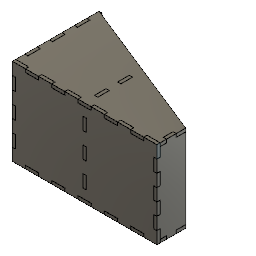
verkefni2_box (Autodesk Fusion 360 design; units mm, degrees)
Autodesk Fusion 360 part; units mm, degrees
sketch "Sketch1" plane through (0, 0, 0) normal (0, 0, 1) x (1, 0, 0)
  line L0 (0, 0) -> (125, 0)
  line L1 (125, 0) -> (125, 75)
  line L2 (125, 75) -> (0, 75)
  line L3 (0, 75) -> (0, 0)
  dimension "d18" = 125
  dimension "d19" = 75
  constraint horizontal L0
  constraint vertical L1
  constraint horizontal L2
  constraint vertical L3
  constraint coincident L0.start L3.end
  measures "d18" distance of L0.start L0.end
  measures "d19" distance of L0.start L2.end
extrude "Extrude1" add sketch "Sketch1" against normal blind 2.8 makes body 1
sketch "Sketch3" plane through (0, 0, 0) normal (-1, 0, 0) x (0, 0, 1)
  line L0 (0, 0) -> (0, 75)
  line L1 (0, 75) -> (-2.8, 75)
  line L2 (-2.8, 75) -> (-2.8, 0)
  line L3 (-2.8, 0) -> (0, 0)
  line L4 (0, 10.7143) -> (-2.8, 10.7143)
  line L5 (-2.8, 10.7143) -> (-2.8, 21.4286)
  line L6 (-2.8, 21.4286) -> (0, 21.4286)
  line L7 (0, 21.4286) -> (0, 10.7143)
  dimension "d24" = 10.7143
  dimension "d25" = 10.7143
  constraint horizontal L4
  constraint vertical L5
  constraint horizontal L6
  constraint vertical L7
  constraint coincident L2 L5.end
  constraint coincident L0 L4.start
  measures "d24" distance of L4.start L6.end
  measures "d25" distance of L0.start L4
extrude "Extrude2" cut sketch "Sketch3" against normal blind 2.8 contours L0 L2 L4 L5 L6 L7 bodies 1
pattern_linear "R-Pattern1" count 3 spacing 21.4286 along (0, 1, 0) of "Extrude2"
sketch "Sketch4" plane through (125, 0, 0) normal (1, 0, 0) x (0, 0, -1)
  line L0 (0, 75) -> (0, 0)
  line L1 (0, 0) -> (2.8, 0)
  line L2 (2.8, 0) -> (2.8, 75)
  line L3 (2.8, 75) -> (0, 75)
  line L4 (2.8, 10.7143) -> (0, 10.7143)
  line L5 (0, 10.7143) -> (0, 21.4286)
  line L6 (0, 21.4286) -> (2.8, 21.4286)
  line L7 (2.8, 21.4286) -> (2.8, 10.7143)
  dimension "d32" = 10.7143
  dimension "d33" = 10.7143
  constraint horizontal L4
  constraint vertical L5
  constraint horizontal L6
  constraint vertical L7
  constraint coincident L0 L5.end
  constraint coincident L2 L4.start
  measures "d32" distance of L4.end L5.end
  measures "d33" distance of L0.end L4
extrude "Extrude3" cut sketch "Sketch4" against normal blind 2.8 contours L0 L2 L4 L5 L6 L7 bodies 1
pattern_linear "R-Pattern2" count 3 spacing 21.4286 along (0, 1, 0) of "Extrude3"
sketch "Sketch5" plane through (0, 0, 0) normal (0, -1, 0) x (1, 0, 0)
  line L0 (125, 0) -> (0, 0)
  line L1 (0, 0) -> (0, -2.8)
  line L2 (0, -2.8) -> (125, -2.8)
  line L3 (125, -2.8) -> (125, 0)
  line L4 (11.3636, 0) -> (22.7273, 0)
  line L5 (22.7273, 0) -> (22.7273, -2.8)
  line L6 (22.7273, -2.8) -> (11.3636, -2.8)
  line L7 (11.3636, -2.8) -> (11.3636, 0)
  dimension "d40" = 11.3636
  dimension "d41" = 11.3636
  constraint horizontal L4
  constraint vertical L5
  constraint horizontal L6
  constraint vertical L7
  constraint coincident L2 L5.end
  constraint coincident L0 L4.start
  measures "d40" distance of L5.end L6.end
  measures "d41" horizontal distance of L0.end L6.end
extrude "Extrude4" cut sketch "Sketch5" against normal blind 2.8 contours L0 L2 L4 L5 L6 L7 bodies 1
pattern_linear "R-Pattern3" count 5 spacing 22.7273 along (1, 0, 0) of "Extrude4"
sketch "Sketch6" plane through (0, 75, 0) normal (0, 1, 0) x (-1, 0, 0)
  line L0 (0, 0) -> (-125, 0)
  line L1 (-125, 0) -> (-125, -2.8)
  line L2 (-125, -2.8) -> (0, -2.8)
  line L3 (0, -2.8) -> (0, 0)
  line L4 (-11.3636, -2.8) -> (-22.7273, -2.8)
  line L5 (-22.7273, -2.8) -> (-22.7273, 0)
  line L6 (-22.7273, 0) -> (-11.3636, 0)
  line L7 (-11.3636, 0) -> (-11.3636, -2.8)
  dimension "d48" = 11.3636
  dimension "d49" = 11.3636
  constraint horizontal L4
  constraint vertical L5
  constraint horizontal L6
  constraint vertical L7
  constraint coincident L0 L5.end
  constraint coincident L2 L4.start
  measures "d48" distance of L4.start L4.end
  measures "d49" distance of L0.start L6.end
extrude "Extrude5" cut sketch "Sketch6" against normal blind 2.8 contours L0 L2 L4 L5 L6 L7 bodies 1
pattern_linear "R-Pattern4" count 5 spacing 22.7273 along (1, 0, 0) of "Extrude5"
sketch "Sketch7" plane through (0, 0, -2.8) normal (0, 0, -1) x (-1, 0, 0)
  line L0 (-102.2727, 75) -> (-102.2727, 72.2)
  line L1 (-102.2727, 72.2) -> (-113.6364, 72.2)
  line L2 (-113.6364, 72.2) -> (-113.6364, 75)
  line L3 (-113.6364, 75) -> (-125, 75)
  line L4 (-125, 75) -> (-125, 64.2857)
  line L5 (-125, 64.2857) -> (-122.2, 64.2857)
  line L6 (-122.2, 64.2857) -> (-122.2, 53.5714)
  line L7 (-122.2, 53.5714) -> (-125, 53.5714)
  line L8 (-125, 53.5714) -> (-125, 42.8571)
  line L9 (-125, 42.8571) -> (-122.2, 42.8571)
  line L10 (-122.2, 42.8571) -> (-122.2, 32.1429)
  line L11 (-122.2, 32.1429) -> (-125, 32.1429)
  line L12 (-125, 32.1429) -> (-125, 21.4286)
  line L13 (-125, 21.4286) -> (-122.2, 21.4286)
  line L14 (-122.2, 21.4286) -> (-122.2, 10.7143)
  line L15 (-122.2, 10.7143) -> (-125, 10.7143)
  line L16 (-125, 10.7143) -> (-125, 0)
  line L17 (-125, 0) -> (-113.6364, 0)
  line L18 (-113.6364, 0) -> (-113.6364, 2.8)
  line L19 (-113.6364, 2.8) -> (-102.2727, 2.8)
  line L20 (-102.2727, 2.8) -> (-102.2727, 0)
  line L21 (-102.2727, 0) -> (-90.9091, 0)
  line L22 (-90.9091, 0) -> (-90.9091, 2.8)
  line L23 (-90.9091, 2.8) -> (-79.5455, 2.8)
  line L24 (-79.5455, 2.8) -> (-79.5455, 0)
  line L25 (-79.5455, 0) -> (-68.1818, 0)
  line L26 (-68.1818, 0) -> (-68.1818, 2.8)
  line L27 (-68.1818, 2.8) -> (-56.8182, 2.8)
  line L28 (-56.8182, 2.8) -> (-56.8182, 0)
  line L29 (-56.8182, 0) -> (-45.4545, 0)
  line L30 (-45.4545, 0) -> (-45.4545, 2.8)
  line L31 (-45.4545, 2.8) -> (-34.0909, 2.8)
  line L32 (-34.0909, 2.8) -> (-34.0909, 0)
  line L33 (-34.0909, 0) -> (-22.7273, 0)
  line L34 (-22.7273, 0) -> (-22.7273, 2.8)
  line L35 (-22.7273, 2.8) -> (-11.3636, 2.8)
  line L36 (-11.3636, 2.8) -> (-11.3636, 0)
  line L37 (-11.3636, 0) -> (0, 0)
  line L38 (0, 0) -> (0, 10.7143)
  line L39 (0, 10.7143) -> (-2.8, 10.7143)
  line L40 (-2.8, 10.7143) -> (-2.8, 21.4286)
  line L41 (-2.8, 21.4286) -> (0, 21.4286)
  line L42 (0, 21.4286) -> (0, 32.1429)
  line L43 (0, 32.1429) -> (-2.8, 32.1429)
  line L44 (-2.8, 32.1429) -> (-2.8, 42.8571)
  line L45 (-2.8, 42.8571) -> (0, 42.8571)
  line L46 (0, 42.8571) -> (0, 53.5714)
  line L47 (0, 53.5714) -> (-2.8, 53.5714)
  line L48 (-2.8, 53.5714) -> (-2.8, 64.2857)
  line L49 (-2.8, 64.2857) -> (0, 64.2857)
  line L50 (0, 64.2857) -> (0, 75)
  line L51 (0, 75) -> (-11.3636, 75)
  line L52 (-11.3636, 75) -> (-11.3636, 72.2)
  line L53 (-11.3636, 72.2) -> (-22.7273, 72.2)
  line L54 (-22.7273, 72.2) -> (-22.7273, 75)
  line L55 (-22.7273, 75) -> (-34.0909, 75)
  line L56 (-34.0909, 75) -> (-34.0909, 72.2)
  line L57 (-34.0909, 72.2) -> (-45.4545, 72.2)
  line L58 (-45.4545, 72.2) -> (-45.4545, 75)
  line L59 (-45.4545, 75) -> (-56.8182, 75)
  line L60 (-56.8182, 75) -> (-56.8182, 72.2)
  line L61 (-56.8182, 72.2) -> (-68.1818, 72.2)
  line L62 (-68.1818, 72.2) -> (-68.1818, 75)
  line L63 (-68.1818, 75) -> (-79.5455, 75)
  line L64 (-79.5455, 75) -> (-79.5455, 72.2)
  line L65 (-79.5455, 72.2) -> (-90.9091, 72.2)
  line L66 (-90.9091, 72.2) -> (-90.9091, 75)
  line L67 (-90.9091, 75) -> (-102.2727, 75)
  line L68 (0, 0) -> (-61.1, 0)
  line L69 (-61.1, 0) -> (-61.1, 75)
  line L70 (-61.1, 0) -> (-63.9, 0)
  line L71 (-63.9, 0) -> (-63.9, 75)
  line L72 (-63.9, 75) -> (-61.1, 75)
  line L73 (-61.1, 75) -> (-61.1, 0)
  line L74 (-61.1, 10.7143) -> (-63.9, 10.7143)
  line L75 (-63.9, 10.7143) -> (-63.9, 21.4286)
  line L76 (-63.9, 21.4286) -> (-61.1, 21.4286)
  line L77 (-61.1, 21.4286) -> (-61.1, 10.7143)
  dimension "d56" = 61.1
  dimension "d57" = 75
  dimension "d58" = 2.8
  dimension "d59" = 75
  dimension "d60" = 10.7143
  dimension "d61" = 10.7143
  constraint coincident L37.end L38.start
  constraint perpendicular L28 L68
  constraint perpendicular L61 L69
  constraint horizontal L70
  constraint vertical L71
  constraint horizontal L72
  constraint vertical L73
  constraint horizontal L74
  constraint vertical L75
  constraint horizontal L76
  constraint vertical L77
  constraint coincident L71 L75.end
  constraint coincident L69 L74.start
  measures "d56" distance of L37.end L68.end
  measures "d57" distance of L68.end L69.end
  measures "d58" distance of L68.end L70.end
  measures "d59" distance of L68.end L69.end
  measures "d60" distance of L70 L74
  measures "d61" distance of L74.end L75.end
extrude "Extrude6" cut sketch "Sketch7" against normal blind 2.8 contours L69 L71 L73 L74 L75 L76 L77 bodies 1
pattern_linear "R-Pattern5" count 3 spacing 21.4286 along (0, 1, 0) of "Extrude6"
sketch "Sketch10" plane through (0, 0, -2.8) normal (0, 0, -1) x (-1, 0, 0)
  line L0 (-63.9, 53.5714) -> (-63.9, 64.2857)
  line L1 (-63.9, 64.2857) -> (-61.1, 64.2857)
  line L2 (-61.1, 64.2857) -> (-61.1, 53.5714)
  line L3 (-61.1, 53.5714) -> (-63.9, 53.5714)
  line L4 (-63.9, 32.1429) -> (-63.9, 42.8571)
  line L5 (-63.9, 42.8571) -> (-61.1, 42.8571)
  line L6 (-61.1, 42.8571) -> (-61.1, 32.1429)
  line L7 (-61.1, 32.1429) -> (-63.9, 32.1429)
  line L8 (-63.9, 10.7143) -> (-63.9, 21.4286)
  line L9 (-63.9, 21.4286) -> (-61.1, 21.4286)
  line L10 (-61.1, 21.4286) -> (-61.1, 10.7143)
  line L11 (-61.1, 10.7143) -> (-63.9, 10.7143)
  line L12 (-102.2727, 75) -> (-102.2727, 72.2)
  line L13 (-102.2727, 72.2) -> (-113.6364, 72.2)
  line L14 (-113.6364, 72.2) -> (-113.6364, 75)
  line L15 (-113.6364, 75) -> (-125, 75)
  line L16 (-125, 75) -> (-125, 64.2857)
  line L17 (-125, 64.2857) -> (-122.2, 64.2857)
  line L18 (-122.2, 64.2857) -> (-122.2, 53.5714)
  line L19 (-122.2, 53.5714) -> (-125, 53.5714)
  line L20 (-125, 53.5714) -> (-125, 42.8571)
  line L21 (-125, 42.8571) -> (-122.2, 42.8571)
  line L22 (-122.2, 42.8571) -> (-122.2, 32.1429)
  line L23 (-122.2, 32.1429) -> (-125, 32.1429)
  line L24 (-125, 32.1429) -> (-125, 21.4286)
  line L25 (-125, 21.4286) -> (-122.2, 21.4286)
  line L26 (-122.2, 21.4286) -> (-122.2, 10.7143)
  line L27 (-122.2, 10.7143) -> (-125, 10.7143)
  line L28 (-125, 10.7143) -> (-125, 0)
  line L29 (-125, 0) -> (-113.6364, 0)
  line L30 (-113.6364, 0) -> (-113.6364, 2.8)
  line L31 (-113.6364, 2.8) -> (-102.2727, 2.8)
  line L32 (-102.2727, 2.8) -> (-102.2727, 0)
  line L33 (-102.2727, 0) -> (-90.9091, 0)
  line L34 (-90.9091, 0) -> (-90.9091, 2.8)
  line L35 (-90.9091, 2.8) -> (-79.5455, 2.8)
  line L36 (-79.5455, 2.8) -> (-79.5455, 0)
  line L37 (-79.5455, 0) -> (-68.1818, 0)
  line L38 (-68.1818, 0) -> (-68.1818, 2.8)
  line L39 (-68.1818, 2.8) -> (-56.8182, 2.8)
  line L40 (-56.8182, 2.8) -> (-56.8182, 0)
  line L41 (-56.8182, 0) -> (-45.4545, 0)
  line L42 (-45.4545, 0) -> (-45.4545, 2.8)
  line L43 (-45.4545, 2.8) -> (-34.0909, 2.8)
  line L44 (-34.0909, 2.8) -> (-34.0909, 0)
  line L45 (-34.0909, 0) -> (-22.7273, 0)
  line L46 (-22.7273, 0) -> (-22.7273, 2.8)
  line L47 (-22.7273, 2.8) -> (-11.3636, 2.8)
  line L48 (-11.3636, 2.8) -> (-11.3636, 0)
  line L49 (-11.3636, 0) -> (0, 0)
  line L50 (0, 0) -> (0, 10.7143)
  line L51 (0, 10.7143) -> (-2.8, 10.7143)
  line L52 (-2.8, 10.7143) -> (-2.8, 21.4286)
  line L53 (-2.8, 21.4286) -> (0, 21.4286)
  line L54 (0, 21.4286) -> (0, 32.1429)
  line L55 (0, 32.1429) -> (-2.8, 32.1429)
  line L56 (-2.8, 32.1429) -> (-2.8, 42.8571)
  line L57 (-2.8, 42.8571) -> (0, 42.8571)
  line L58 (0, 42.8571) -> (0, 53.5714)
  line L59 (0, 53.5714) -> (-2.8, 53.5714)
  line L60 (-2.8, 53.5714) -> (-2.8, 64.2857)
  line L61 (-2.8, 64.2857) -> (0, 64.2857)
  line L62 (0, 64.2857) -> (0, 75)
  line L63 (0, 75) -> (-11.3636, 75)
  line L64 (-11.3636, 75) -> (-11.3636, 72.2)
  line L65 (-11.3636, 72.2) -> (-22.7273, 72.2)
  line L66 (-22.7273, 72.2) -> (-22.7273, 75)
  line L67 (-22.7273, 75) -> (-34.0909, 75)
  line L68 (-34.0909, 75) -> (-34.0909, 72.2)
  line L69 (-34.0909, 72.2) -> (-45.4545, 72.2)
  line L70 (-45.4545, 72.2) -> (-45.4545, 75)
  line L71 (-45.4545, 75) -> (-56.8182, 75)
  line L72 (-56.8182, 75) -> (-56.8182, 72.2)
  line L73 (-56.8182, 72.2) -> (-68.1818, 72.2)
  line L74 (-68.1818, 72.2) -> (-68.1818, 75)
  line L75 (-68.1818, 75) -> (-79.5455, 75)
  line L76 (-79.5455, 75) -> (-79.5455, 72.2)
  line L77 (-79.5455, 72.2) -> (-90.9091, 72.2)
  line L78 (-90.9091, 72.2) -> (-90.9091, 75)
  line L79 (-90.9091, 75) -> (-102.2727, 75)
  line L80 (0, 0) -> (-61.1, 0)
  line L81 (-61.1, 0) -> (-63.9, 0)
  line L82 (-63.9, 0) -> (-63.9, 75)
  line L83 (-63.9, 75) -> (-61.1, 75)
  line L84 (-61.1, 75) -> (-61.1, 0)
  dimension "d72" = 61.1
  dimension "d73" = 2.8
  dimension "d74" = 75
  constraint coincident L49.end L50.start
  constraint perpendicular L50 L80
  constraint horizontal L81
  constraint vertical L82
  constraint horizontal L83
  constraint vertical L84
  measures "d72" distance of L49.end L80.end
  measures "d73" distance of L80.end L81.end
  measures "d74" distance of L80.end L83.end
extrude "Extrude7" add sketch "Sketch10" along normal blind 47.2 separate body contours L0 L1 L2 L3 L82 L84 | L3 L5 L82 L84 | L1 L73 L82 L84 | L4 L5 L6 L7 L82 L84 | L73 L82 L83 L84 | L7 L9 L82 L84 | L8 L9 L10 L11 L82 L84 | L11 L39 L82 L84 | L39 L81 L82 L84 makes body 2
sketch "Sketch12" plane through (0, 0, -2.8) normal (0, 0, 1) x (1, 0, 0)
  line L0 (63.9, 75) -> (61.1, 75)
  line L1 (61.1, 75) -> (61.1, 0)
  line L2 (61.1, 0) -> (63.9, 0)
  line L3 (63.9, 0) -> (63.9, 75)
  line L4 (61.1, 64.2857) -> (63.9, 64.2857)
  line L5 (63.9, 64.2857) -> (63.9, 53.5714)
  line L6 (63.9, 53.5714) -> (61.1, 53.5714)
  line L7 (61.1, 53.5714) -> (61.1, 64.2857)
  dimension "d81" = 10.7143
  dimension "d82" = 10.7143
  constraint horizontal L4
  constraint vertical L5
  constraint horizontal L6
  constraint vertical L7
  constraint coincident L3 L5.end
  constraint coincident L1 L4.start
  measures "d81" distance of L4.start L6.end
  measures "d82" distance of L0.end L4
extrude "Extrude8" add sketch "Sketch12" along normal blind 2.8 contours L1 L3 L4 L5 L6 L7 bodies 2
pattern_linear "R-Pattern6" count 3 spacing 21.4286 along (0, -1, 0) of "Extrude8"
sketch "Sketch13" plane through (0, 0, -50) normal (0, 0, -1) x (-1, 0, 0)
  line L0 (-61.1, 75) -> (-63.9, 75)
  line L1 (-63.9, 75) -> (-63.9, 0)
  line L2 (-63.9, 0) -> (-61.1, 0)
  line L3 (-61.1, 0) -> (-61.1, 75)
  line L4 (-61.1, 0) -> (-63.9, 0)
  line L5 (-63.9, 0) -> (-63.9, 2.8)
  line L6 (-63.9, 2.8) -> (-61.1, 2.8)
  line L7 (-61.1, 2.8) -> (-61.1, 0)
  dimension "d89" = 2.8
  dimension "d90" = 2.8
  constraint horizontal L4
  constraint vertical L5
  constraint horizontal L6
  constraint vertical L7
  constraint coincident L2.end L3.start
  measures "d89" distance of L2.end L1.end
  measures "d90" distance of L2.end L6.end
extrude "Extrude9" cut sketch "Sketch13" against normal blind 47.2 contours L1 L2 L3 L4 L5 L6 L7 bodies 2
sketch "Sketch14" plane through (0, 0, -50) normal (0, 0, -1) x (-1, 0, 0)
  line L0 (-63.9, 2.8) -> (-61.1, 2.8)
  line L1 (-61.1, 2.8) -> (-61.1, 75)
  line L2 (-61.1, 75) -> (-63.9, 75)
  line L3 (-63.9, 75) -> (-63.9, 2.8)
  line L4 (-61.1, 75) -> (-63.9, 75)
  line L5 (-63.9, 75) -> (-63.9, 72.2)
  line L6 (-63.9, 72.2) -> (-61.1, 72.2)
  line L7 (-61.1, 72.2) -> (-61.1, 75)
  dimension "d93" = 2.8
  dimension "d94" = 2.8
  constraint horizontal L4
  constraint vertical L5
  constraint horizontal L6
  constraint vertical L7
  constraint coincident L1.end L2.start
  measures "d93" distance of L1.end L2.end
  measures "d94" distance of L1.end L6.end
extrude "Extrude10" cut sketch "Sketch14" against normal blind 47.2 contours L1 L2 L3 L4 L5 L6 L7 bodies 2
sketch "Sketch15" plane through (0, 2.8, 0) normal (0, -1, 0) x (1, 0, 0)
  line L0 (61.1, -50) -> (63.9, -50)
  line L1 (63.9, -50) -> (63.9, -2.8)
  line L2 (63.9, -2.8) -> (61.1, -2.8)
  line L3 (61.1, -2.8) -> (61.1, -50)
  line L4 (63.9, -40) -> (61.1, -40)
  line L5 (61.1, -40) -> (61.1, -30)
  line L6 (61.1, -30) -> (63.9, -30)
  line L7 (63.9, -30) -> (63.9, -40)
  dimension "d97" = 10
  dimension "d98" = 10
  constraint horizontal L4
  constraint vertical L5
  constraint horizontal L6
  constraint vertical L7
  constraint coincident L3 L5.end
  constraint coincident L1 L4.start
  measures "d97" distance of L4.start L6.end
  measures "d98" distance of L0.end L4
extrude "Extrude11" add sketch "Sketch15" along normal blind 2.8 contours L1 L3 L4 L5 L6 L7 bodies 2
pattern_linear "R-Pattern7" count 2 spacing 20 along (0, 0, 1) of "Extrude11"
sketch "Sketch16" plane through (0, 72.2, 0) normal (0, 1, 0) x (-1, 0, 0)
  line L0 (-63.9, -50) -> (-61.1, -50)
  line L1 (-61.1, -50) -> (-61.1, -2.8)
  line L2 (-61.1, -2.8) -> (-63.9, -2.8)
  line L3 (-63.9, -2.8) -> (-63.9, -50)
  line L4 (-61.1, -40) -> (-63.9, -40)
  line L5 (-63.9, -40) -> (-63.9, -30)
  line L6 (-63.9, -30) -> (-61.1, -30)
  line L7 (-61.1, -30) -> (-61.1, -40)
  dimension "d105" = 10
  dimension "d106" = 10
  constraint horizontal L4
  constraint vertical L5
  constraint horizontal L6
  constraint vertical L7
  constraint coincident L3 L5.end
  constraint coincident L1 L4.start
  measures "d105" distance of L4.start L6.end
  measures "d106" distance of L0.end L4
extrude "Extrude12" add sketch "Sketch16" along normal blind 2.8 contours L1 L3 L4 L5 L6 L7 bodies 2
pattern_linear "R-Pattern8" count 2 spacing 20 along (0, 0, 1) of "Extrude12"
sketch "Sketch17" plane through (0, 75, 0) normal (0, 1, 0) x (-1, 0, 0)
  line L0 (-11.3636, 0) -> (-11.3636, -2.8)
  line L1 (-11.3636, -2.8) -> (0, -2.8)
  line L2 (0, -2.8) -> (0, 0)
  line L3 (0, 0) -> (-11.3636, 0)
  line L4 (0, 0) -> (-125, 0)
  line L5 (0, 0) -> (0, -75)
  line L6 (-125, 0) -> (-125, -25)
  line L7 (0, -75) -> (-125, -25)
  line L8 (0, 0) -> (-61.1, 0)
  line L9 (-61.1, 0) -> (-63.9, 0)
  line L10 (-63.9, 0) -> (-63.9, -50)
  line L11 (-63.9, -50) -> (-61.1, -50)
  line L12 (-61.1, -50) -> (-61.1, 0)
  line L13 (-61.1, -50) -> (-63.9, -50)
  line L14 (-63.9, -50) -> (-63.9, -40)
  line L15 (-63.9, -40) -> (-61.1, -40)
  line L16 (-61.1, -40) -> (-61.1, -50)
  line L17 (-61.1, -40) -> (-63.9, -40)
  line L18 (-63.9, -40) -> (-63.9, -30)
  line L19 (-63.9, -30) -> (-61.1, -30)
  line L20 (-61.1, -30) -> (-61.1, -40)
  line L21 (-61.1, -30) -> (-63.9, -30)
  line L22 (-63.9, -30) -> (-63.9, -20)
  line L23 (-63.9, -20) -> (-61.1, -20)
  line L24 (-61.1, -20) -> (-61.1, -30)
  line L25 (-61.1, -20) -> (-63.9, -20)
  line L26 (-63.9, -20) -> (-63.9, -10)
  line L27 (-63.9, -10) -> (-61.1, -10)
  line L28 (-61.1, -10) -> (-61.1, -20)
  line L29 (-61.1, -10) -> (-63.9, -10)
  line L30 (-63.9, -10) -> (-63.9, -20)
  line L31 (-63.9, -20) -> (-61.1, -20)
  line L32 (-61.1, -20) -> (-61.1, -10)
  line L33 (-61.1, -10) -> (-63.9, -10)
  line L34 (-63.9, -10) -> (-63.9, 0)
  line L35 (-63.9, 0) -> (-61.1, 0)
  line L36 (-61.1, 0) -> (-61.1, -10)
  dimension "d113" = 125
  dimension "d114" = 75
  dimension "d115" = 25
  dimension "d116" = 134.6291
  dimension "d117" = 61.1
  dimension "d118" = 2.8
  dimension "d119" = 50
  dimension "d120" = 2.8
  dimension "d121" = 10
  dimension "d122" = 2.8
  dimension "d123" = 10
  dimension "d124" = 2.8
  dimension "d125" = 10
  dimension "d126" = 2.8
  dimension "d127" = 10
  dimension "d128" = 2.8
  dimension "d129" = 10
  dimension "d130" = 2.8
  dimension "d131" = 10
  constraint coincident L2.end L3.start
  constraint perpendicular L2 L4
  constraint perpendicular L3 L5
  constraint perpendicular L4 L6
  constraint perpendicular L2 L8
  constraint horizontal L9
  constraint vertical L10
  constraint horizontal L11
  constraint vertical L12
  constraint horizontal L13
  constraint vertical L14
  constraint horizontal L15
  constraint vertical L16
  constraint horizontal L17
  constraint vertical L18
  constraint horizontal L19
  constraint vertical L20
  constraint horizontal L21
  constraint vertical L22
  constraint horizontal L23
  constraint vertical L24
  constraint horizontal L25
  constraint vertical L26
  constraint horizontal L27
  constraint vertical L28
  constraint horizontal L29
  constraint vertical L30
  constraint horizontal L31
  constraint vertical L32
  constraint horizontal L33
  constraint vertical L34
  constraint horizontal L35
  constraint vertical L36
  measures "d113" distance of L2.end L4.end
  measures "d114" distance of L2.end L5.end
  measures "d115" distance of L4.end L6.end
  measures "d116" distance of L5.end L6.end
  measures "d117" distance of L2.end L8.end
  measures "d118" distance of L8.end L9.end
  measures "d119" distance of L8.end L11.end
  measures "d120" distance of L11.end L10.end
  measures "d121" distance of L11.end L15.end
  measures "d122" distance of L15.end L14.end
  measures "d123" distance of L15.end L19.end
  measures "d124" distance of L19.end L18.end
  measures "d125" distance of L19.end L23.end
  measures "d126" distance of L23.end L22.end
  measures "d127" distance of L23.end L27.end
  measures "d128" distance of L27.end L26.end
  measures "d129" distance of L27.end L23.end
  measures "d130" distance of L27.end L26.end
  measures "d131" distance of L27.end L8.end
extrude "Extrude13" add sketch "Sketch17" against normal blind 2.8 separate body contours L0 L1 L4 L5 L7 L8 L11 L12 L13 L16 L20 L24 L28 L32 L36 | L4 L9 L10 L12 L27 L29 L33 L34 L35 L36 | L4 L6 L7 L10 L14 L18 L22 L26 L30 L34 | L10 L12 L19 L21 L22 L23 L24 L25 L31 | L7 L10 L11 L12 L13 L14 L15 L16 L17 makes body 3
combine "Combine1" operation cut target body 3 tool bodies 1 2 keep tools
sketch "Sketch18" plane through (0, 0, 0) normal (0, -1, 0) x (1, 0, 0)
  line L0 (113.6364, 0) -> (113.6364, -2.8)
  line L1 (113.6364, -2.8) -> (125, -2.8)
  line L2 (125, -2.8) -> (125, 0)
  line L3 (125, 0) -> (113.6364, 0)
  line L4 (0, 0) -> (125, 0)
  line L5 (125, 0) -> (125, -25)
  line L6 (0, 0) -> (0, -75)
  line L7 (0, -75) -> (125, -25)
  line L8 (125, 0) -> (63.9, 0)
  line L9 (63.9, 0) -> (61.1, 0)
  line L10 (61.1, 0) -> (61.1, -50)
  line L11 (61.1, -50) -> (63.9, -50)
  line L12 (63.9, -50) -> (63.9, 0)
  line L13 (63.9, -50) -> (61.1, -50)
  line L14 (61.1, -50) -> (61.1, -40)
  line L15 (61.1, -40) -> (63.9, -40)
  line L16 (63.9, -40) -> (63.9, -50)
  line L17 (63.9, -40) -> (61.1, -40)
  line L18 (61.1, -40) -> (61.1, -30)
  line L19 (61.1, -30) -> (63.9, -30)
  line L20 (63.9, -30) -> (63.9, -40)
  line L21 (63.9, -30) -> (61.1, -30)
  line L22 (61.1, -30) -> (61.1, -20)
  line L23 (61.1, -20) -> (63.9, -20)
  line L24 (63.9, -20) -> (63.9, -30)
  line L25 (63.9, -20) -> (61.1, -20)
  line L26 (61.1, -20) -> (61.1, -10)
  line L27 (61.1, -10) -> (63.9, -10)
  line L28 (63.9, -10) -> (63.9, -20)
  line L29 (63.9, -10) -> (61.1, -10)
  line L30 (61.1, -10) -> (61.1, 0)
  line L31 (61.1, 0) -> (63.9, 0)
  line L32 (63.9, 0) -> (63.9, -10)
  dimension "d134" = 125
  dimension "d135" = 25
  dimension "d136" = 75
  dimension "d137" = 134.6291
  dimension "d138" = 61.1
  dimension "d139" = 2.8
  dimension "d140" = 50
  dimension "d141" = 2.8
  dimension "d142" = 10
  dimension "d143" = 2.8
  dimension "d144" = 10
  dimension "d145" = 2.8
  dimension "d146" = 10
  dimension "d147" = 2.8
  dimension "d148" = 10
  dimension "d149" = 2.8
  dimension "d150" = 10
  constraint coincident L4.start L6.start
  constraint coincident L2.end L3.start
  constraint perpendicular L4 L5
  constraint perpendicular L4 L6
  constraint perpendicular L0 L8
  constraint horizontal L9
  constraint vertical L10
  constraint horizontal L11
  constraint vertical L12
  constraint horizontal L13
  constraint vertical L14
  constraint horizontal L15
  constraint vertical L16
  constraint horizontal L17
  constraint vertical L18
  constraint horizontal L19
  constraint vertical L20
  constraint horizontal L21
  constraint vertical L22
  constraint horizontal L23
  constraint vertical L24
  constraint horizontal L25
  constraint vertical L26
  constraint horizontal L27
  constraint vertical L28
  constraint horizontal L29
  constraint vertical L30
  constraint horizontal L31
  constraint vertical L32
  measures "d134" distance of L4.start L2.end
  measures "d135" distance of L2.end L5.end
  measures "d136" distance of L4.start L6.end
  measures "d137" distance of L6.end L5.end
  measures "d138" distance of L2.end L8.end
  measures "d139" distance of L8.end L9.end
  measures "d140" distance of L8.end L11.end
  measures "d141" distance of L11.end L10.end
  measures "d142" distance of L11.end L15.end
  measures "d143" distance of L15.end L14.end
  measures "d144" distance of L15.end L19.end
  measures "d145" distance of L19.end L18.end
  measures "d146" distance of L19.end L23.end
  measures "d147" distance of L23.end L22.end
  measures "d148" distance of L23.end L27.end
  measures "d149" distance of L27.end L26.end
  measures "d150" distance of L27.end L8.end
extrude "Extrude14" add sketch "Sketch18" against normal blind 2.8 separate body contours L0 L1 L4 L5 L7 L8 L12 L16 L20 L24 L28 L32 | L4 L9 L10 L12 L27 L29 L30 L31 L32 | L4 L6 L7 L10 L11 L13 L14 L18 L22 L26 L30 | L10 L12 L19 L21 L22 L23 L24 L25 | L7 L10 L11 L12 L13 L14 L15 L16 L17 makes body 4
combine "Combine2" operation cut target body 4 tool bodies 2 1 keep tools
sketch "Sketch19" plane through (125, 0, 0) normal (1, 0, 0) x (0, 0, -1)
  line L0 (0, 64.2857) -> (2.8, 64.2857)
  line L1 (2.8, 64.2857) -> (2.8, 75)
  line L2 (2.8, 75) -> (0, 75)
  line L3 (0, 75) -> (0, 64.2857)
sketch "Sketch20" plane through (125, 0, 0) normal (1, 0, 0) x (0, 0, -1)
  line L0 (2.8, 75) -> (2.8, 72.2)
  line L1 (2.8, 72.2) -> (25, 72.2)
  line L2 (25, 72.2) -> (25, 75)
  line L3 (25, 75) -> (2.8, 75)
  line L4 (16.6667, 75) -> (8.3333, 75)
  line L5 (8.3333, 75) -> (8.3333, 72.2)
  line L6 (8.3333, 72.2) -> (16.6667, 72.2)
  line L7 (16.6667, 72.2) -> (16.6667, 75)
  dimension "d153" = 8.3333
  dimension "d154" = 8.3333
  constraint horizontal L4
  constraint vertical L5
  constraint horizontal L6
  constraint vertical L7
  constraint coincident L1 L5.end
  constraint coincident L3 L4.start
  measures "d153" distance of L4.start L4.end
  measures "d154" distance of L2.end L7
extrude "Extrude15" cut sketch "Sketch20" against normal blind 2.8 contours L1 L3 L4 L5 L6 L7 bodies 3
pattern_linear "R-Pattern9" count 1 spacing 0 along (0, 0, 1) of "Extrude15"
sketch "Sketch21" plane through (125, 0, 0) normal (1, 0, 0) x (0, 0, -1)
  line L0 (2.8, 0) -> (25, 0)
  line L1 (25, 0) -> (25, 2.8)
  line L2 (25, 2.8) -> (2.8, 2.8)
  line L3 (2.8, 2.8) -> (2.8, 0)
  line L4 (16.6667, 2.8) -> (8.3333, 2.8)
  line L5 (8.3333, 2.8) -> (8.3333, 0)
  line L6 (8.3333, 0) -> (16.6667, 0)
  line L7 (16.6667, 0) -> (16.6667, 2.8)
  dimension "d161" = 8.3333
  dimension "d162" = 8.3333
  constraint horizontal L4
  constraint vertical L5
  constraint horizontal L6
  constraint vertical L7
  constraint coincident L0 L5.end
  constraint coincident L2 L4.start
  measures "d161" distance of L5.end L6.end
  measures "d162" distance of L0.end L7
extrude "Extrude16" cut sketch "Sketch21" against normal blind 2.8 contours L0 L2 L4 L5 L6 L7 bodies 4
pattern_linear "R-Pattern10" count 1 spacing 0 along (0, 0, -1) of "Extrude16"
sketch "Sketch22" plane through (125, 0, 0) normal (1, 0, 0) x (0, 0, -1)
  line L0 (16.6667, 75) -> (16.6667, 72.2)
  line L1 (16.6667, 72.2) -> (25, 72.2)
  line L2 (25, 72.2) -> (25, 75)
  line L3 (25, 75) -> (16.6667, 75)
  line L4 (25, 75) -> (0, 75)
  line L5 (0, 75) -> (0, 0)
  line L6 (0, 0) -> (25, 0)
  line L7 (25, 0) -> (25, 75)
  dimension "d169" = 25
  dimension "d170" = 75
  constraint horizontal L4
  constraint vertical L5
  constraint horizontal L6
  constraint vertical L7
  constraint coincident L2.end L3.start
  measures "d169" distance of L2.end L4.end
  measures "d170" distance of L2.end L6.end
extrude "Extrude17" add sketch "Sketch22" against normal blind 2.8 separate body contours L0 L1 L4 L5 L6 L7 makes body 5
combine "Combine3" operation cut target body 5 tool bodies 3 1 4 keep tools
sketch "Sketch23" plane through (0, 0, 0) normal (-1, 0, 0) x (0, 0, 1)
  line L0 (-2.8, 0) -> (-2.8, 2.8)
  line L1 (-2.8, 2.8) -> (-75, 2.8)
  line L2 (-75, 2.8) -> (-75, 0)
  line L3 (-75, 0) -> (-2.8, 0)
  line L4 (-64.2857, 0) -> (-53.5714, 0)
  line L5 (-53.5714, 0) -> (-53.5714, 2.8)
  line L6 (-53.5714, 2.8) -> (-64.2857, 2.8)
  line L7 (-64.2857, 2.8) -> (-64.2857, 0)
  dimension "d173" = 10.7143
  dimension "d174" = 10.7143
  constraint horizontal L4
  constraint vertical L5
  constraint horizontal L6
  constraint vertical L7
  constraint coincident L1 L5.end
  constraint coincident L3 L4.start
  measures "d173" distance of L4.start L4.end
  measures "d174" distance of L2.end L7
extrude "Extrude18" cut sketch "Sketch23" against normal blind 2.8 contours L1 L3 L4 L5 L6 L7 bodies 4
pattern_linear "R-Pattern11" count 3 spacing 21.4286 along (0, 0, 1) of "Extrude18"
sketch "Sketch24" plane through (0, 0, 0) normal (-1, 0, 0) x (0, 0, 1)
  line L0 (-2.8, 75) -> (-75, 75)
  line L1 (-75, 75) -> (-75, 72.2)
  line L2 (-75, 72.2) -> (-2.8, 72.2)
  line L3 (-2.8, 72.2) -> (-2.8, 75)
  line L4 (-64.2857, 72.2) -> (-53.5714, 72.2)
  line L5 (-53.5714, 72.2) -> (-53.5714, 75)
  line L6 (-53.5714, 75) -> (-64.2857, 75)
  line L7 (-64.2857, 75) -> (-64.2857, 72.2)
  dimension "d181" = 10.7143
  dimension "d182" = 10.7143
  constraint horizontal L4
  constraint vertical L5
  constraint horizontal L6
  constraint vertical L7
  constraint coincident L0 L5.end
  constraint coincident L2 L4.start
  measures "d181" distance of L4.start L4.end
  measures "d182" distance of L1.end L7
extrude "Extrude19" cut sketch "Sketch24" against normal blind 2.8 contours L0 L2 L4 L5 L6 L7 bodies 3
pattern_linear "R-Pattern12" count 3 spacing 21.4286 along (0, 0, 1) of "Extrude19"
sketch "Sketch25" plane through (0, 0, 0) normal (-1, 0, 0) x (0, 0, 1)
  line L0 (-64.2857, 0) -> (-64.2857, 2.8)
  line L1 (-64.2857, 2.8) -> (-75, 2.8)
  line L2 (-75, 2.8) -> (-75, 0)
  line L3 (-75, 0) -> (-64.2857, 0)
  line L4 (-75, 0) -> (0, 0)
  line L5 (0, 0) -> (0, 75)
  line L6 (0, 75) -> (-75, 75)
  line L7 (-75, 75) -> (-75, 0)
  dimension "d189" = 75
  dimension "d190" = 75
  constraint horizontal L4
  constraint vertical L5
  constraint horizontal L6
  constraint vertical L7
  constraint coincident L2.end L3.start
  measures "d189" distance of L2.end L4.end
  measures "d190" distance of L4.end L5.end
extrude "Extrude20" add sketch "Sketch25" against normal blind 2.8 separate body contours L0 L1 L4 L5 L6 L7 makes body 6
combine "Combine4" operation cut target body 6 tool bodies 4 3 1 keep tools
equation "lengd = 62.5 * 2 mm"
equation "breidd = 37.5 * 2 mm"
equation "toppur = 37.5 * 2 mm"
equation "botn = 12.5 * 2 mm"
equation "þykkt = 2.8 mm"
equation "f_lengd = 5"
equation "f_breidd = 3"
equation "f_toppur = 3"
equation "f_botn = 1"
equation "f_midja = 2"
equation "f_lengd_f = lengd / ( ( f_lengd * 2 ) + 1 )"
equation "f_breidd_f = breidd / ( ( f_breidd * 2 ) + 1 )"
equation "f_toppur_f = toppur / ( ( f_toppur * 2 ) + 1 )"
equation "f_botn_f = botn / ( ( f_botn * 2 ) + 1 )"
equation "ská = sqrt(( toppur - botn ) ^ 2 + lengd ^ 2)"
equation "midja = toppur - ( toppur - botn ) / 2"
equation "f_midja_F = midja / ( ( f_midja * 2 ) + 1 )"
equation "d18 = lengd"
equation "d19 = breidd"
equation "d20 = -þykkt"
equation "d24 = f_breidd_f"
equation "d25 = f_breidd_f"
equation "d26 = -þykkt"
equation "d28 = f_breidd"
equation "d30 = breidd - f_breidd_f * 3"
equation "d32 = f_breidd_f"
equation "d33 = f_breidd_f"
equation "d34 = -þykkt"
equation "d36 = f_breidd"
equation "d38 = -( breidd - f_breidd_f * 3 )"
equation "d40 = f_lengd_f"
equation "d41 = f_lengd_f"
equation "d42 = -þykkt"
equation "d44 = f_lengd"
equation "d46 = -( lengd - f_lengd_f * 3 )"
equation "d48 = f_lengd_f"
equation "d49 = f_lengd_f"
equation "d50 = -þykkt"
equation "d52 = f_lengd"
equation "d54 = -( lengd - 3 * f_lengd_f )"
equation "d56 = lengd / 2 - þykkt / 2"
equation "d57 = breidd"
equation "d58 = þykkt"
equation "d59 = breidd"
equation "d60 = f_breidd_f"
equation "d61 = f_breidd_f"
equation "d62 = -þykkt"
equation "d64 = f_breidd"
equation "d66 = -( breidd - f_breidd_f * 3 )"
equation "d72 = lengd / 2 - þykkt / 2"
equation "d73 = þykkt"
equation "d74 = breidd"
equation "d75 = midja - þykkt"
equation "d81 = f_breidd_f"
equation "d82 = f_breidd_f"
equation "d83 = þykkt"
equation "d85 = f_breidd"
equation "d87 = -( breidd - f_breidd_f * 3 )"
equation "d89 = þykkt"
equation "d90 = þykkt"
equation "d91 = -( midja - þykkt )"
equation "d93 = þykkt"
equation "d94 = þykkt"
equation "d95 = -( midja - þykkt )"
equation "d97 = f_midja_F"
equation "d98 = f_midja_F"
equation "d99 = þykkt"
equation "d101 = f_midja"
equation "d103 = midja - f_midja_F * 3"
equation "d105 = f_midja_F"
equation "d106 = f_midja_F"
equation "d107 = þykkt"
equation "d109 = f_midja"
equation "d111 = -( midja - f_midja_F * 3 )"
equation "d113 = lengd"
equation "d114 = toppur"
equation "d115 = botn"
equation "d116 = ská"
equation "d117 = lengd / 2 - þykkt / 2"
equation "d118 = þykkt"
equation "d119 = midja"
equation "d120 = þykkt"
equation "d121 = f_midja_F"
equation "d122 = þykkt"
equation "d123 = f_midja_F"
equation "d124 = þykkt"
equation "d125 = f_midja_F"
equation "d126 = þykkt"
equation "d127 = f_midja_F"
equation "d128 = þykkt"
equation "d129 = f_midja_F"
equation "d130 = þykkt"
equation "d131 = f_midja_F"
equation "d132 = -þykkt"
equation "d134 = lengd"
equation "d135 = botn"
equation "d136 = toppur"
equation "d137 = ská"
equation "d138 = lengd / 2 - þykkt / 2"
equation "d139 = þykkt"
equation "d140 = midja"
equation "d141 = þykkt"
equation "d142 = f_midja_F"
equation "d143 = þykkt"
equation "d144 = f_midja_F"
equation "d145 = þykkt"
equation "d146 = f_midja_F"
equation "d147 = þykkt"
equation "d148 = f_midja_F"
equation "d149 = þykkt"
equation "d150 = f_midja_F"
equation "d151 = -þykkt"
equation "d153 = f_botn_f"
equation "d154 = f_botn_f"
equation "d155 = -þykkt"
equation "d157 = f_botn"
equation "d159 = botn - f_botn_f * 3"
equation "d161 = f_botn_f"
equation "d162 = f_botn_f"
equation "d163 = -þykkt"
equation "d165 = f_botn"
equation "d167 = -( botn - f_botn_f * 3 )"
equation "d169 = botn"
equation "d170 = breidd"
equation "d171 = -þykkt"
equation "d173 = f_toppur_f"
equation "d174 = f_toppur_f"
equation "d175 = -þykkt"
equation "d177 = f_toppur"
equation "d179 = toppur - 3 * f_toppur_f"
equation "d181 = f_toppur_f"
equation "d182 = f_toppur_f"
equation "d183 = -þykkt"
equation "d185 = f_toppur"
equation "d187 = -( toppur - 3 * f_toppur_f )"
equation "d189 = toppur"
equation "d190 = breidd"
equation "d191 = -þykkt"
named bodies: "botn", "Midja", "vh", "hh", "framan", "aftan"
